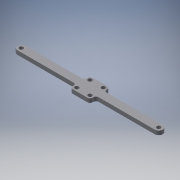
# Autodesk Inventor part: led_brace
Saved by Autodesk Inventor 2017 (Build 210142000, 142)
## iProperties
Created: 2017-06-15
Part Number: led_brace
Material: Generic
Document SubType Name: Modeling
Designer: millerid
Density: 1 g/cm^3
Appearance: Default
Author: millerid
Autodesk Inventor part; units mm, degrees
ref_plane "YZ Plane" through (0, 0, 0) normal (1, 0, 0) x (0, 1, 0)
ref_plane "XZ Plane" through (0, 0, 0) normal (0, 1, 0) x (-1, 0, 0)
ref_plane "XY Plane" through (0, 0, 0) normal (0, 0, 1) x (1, 0, 0)
sketch "Sketch1" plane through (0, 0, 0) normal (0, 1, 0) x (-1, 0, 0)
  circle A0 centre (13.6692, 0.0318) radius 1.5
  circle A1 centre (-89.8308, 0.0318) radius 1.5
  arc A2 (13.1692, -3) -> (14.1692, 2.9161) centre (13.6692, -0.042) ccw
  arc A3 (-89.8308, 3) -> (-89.8308, -3) centre (-89.8308, 0) ccw
  line L0 (-32.5808, -7.4682) -> (-43.5808, -7.4682)
  line L1 (-43.5808, 7.5318) -> (-32.5808, 7.5318)
  line L2 (13.1692, -3) -> (-28.5808, -3)
  line L3 (14.1692, 2.9161) -> (-28.5808, 2.9161)
  line L4 (-47.5808, -3) -> (-89.8308, -3)
  line L5 (-89.8308, 3) -> (-47.5808, 3)
  line L6 (-30.5808, -5.4682) -> (-30.5808, -5)
  line L7 (-30.5808, 4.9161) -> (-30.5808, 5.5318)
  line L8 (-45.5808, 5.5318) -> (-45.5808, 5)
  line L9 (-45.5808, -5) -> (-45.5808, -5.4682)
  circle A4 centre (-33.0808, -5.042) radius 1.5
  circle A5 centre (-43.0808, -5.042) radius 1.5
  circle A6 centre (-33.0808, 4.958) radius 1.5
  circle A7 centre (-43.0808, 4.958) radius 1.5
  arc A8 (-28.5808, -3) -> (-30.5808, -5) centre (-28.5808, -5) ccw
  arc A9 (-32.5808, -7.4682) -> (-30.5808, -5.4682) centre (-32.5808, -5.4682) ccw
  arc A10 (-45.5808, -5.4682) -> (-43.5808, -7.4682) centre (-43.5808, -5.4682) ccw
  arc A11 (-45.5808, -5) -> (-47.5808, -3) centre (-47.5808, -5) ccw
  arc A12 (-30.5808, 4.9161) -> (-28.5808, 2.9161) centre (-28.5808, 4.9161) ccw
  arc A13 (-47.5808, 3) -> (-45.5808, 5) centre (-47.5808, 5) ccw
  arc A14 (-43.5808, 7.5318) -> (-45.5808, 5.5318) centre (-43.5808, 5.5318) ccw
  arc A15 (-30.5808, 5.5318) -> (-32.5808, 7.5318) centre (-32.5808, 5.5318) ccw
  point P0 (-45.5808, 7.5318)
  point P1 (-45.5808, -7.4682)
  point P2 (-30.5808, 7.5318)
  dimension "d39" = 3
  dimension "d40" = 3
  dimension "d41" = 103.5
  dimension "d42" = 6
  dimension "d43" = 3
  dimension "d44" = 3
  dimension "d45" = 15
  dimension "d46" = 15
  dimension "d47" = 7.5
  dimension "d49" = 0
  dimension "d50" = 0
  dimension "d51" = 3
  dimension "d52" = 3
  dimension "d53" = 10
  dimension "d54" = 3
  dimension "d55" = 10
  dimension "d56" = 3
  dimension "d57" = 5
  dimension "d58" = 10
  dimension "d59" = 2
  dimension "d62" = 46.75
  dimension "d63" = 46.75
  dimension "d64" = 10
  dimension "d65" = 42.25
  constraints: 20 end point, 20 point on circle, 16 centre point, 16 tangent, 7 equal radius, 6 point on line, 4 collinear, 3 parallel, 2 horizontal, 1 vertical
  measures "d39" diameter of A0
  measures "d40" diameter of A1
  measures "d41" distance of A1.centre A0.centre
  measures "d42" distance of L2.start L3.start
  measures "d43" radius of A2
  measures "d44" radius of A3
  measures "d45" distance of point (-45.581, 7.532) point (-30.581, 7.532)
  measures "d46" distance of point (-45.581, -7.468) point (-45.581, 7.532)
  measures "d47" distance from line of A0.centre L0
  measures "d49" horizontal distance of A2.centre A0.centre
  measures "d50" horizontal distance of A3.centre A1.centre
  measures "d51" diameter of A4
  measures "d52" diameter of A5
  measures "d53" distance of A5.centre A4.centre
  measures "d54" diameter of A6
  measures "d55" distance of A6.centre A4.centre
  measures "d56" diameter of A7
  measures "d57" vertical distance of A2.centre A4.centre
  measures "d58" distance of A5.centre A7.centre
  measures "d59" radius of A8
  measures "d62" horizontal distance of A2.centre A4.centre
  measures "d63" horizontal distance of A0.centre A6.centre
  measures "d64" distance of A7.centre A6.centre
  measures "d65" horizontal distance of A3.centre A11.centre
extrude "Extrusion2" add sketch "Sketch1" along normal blind 3
equation "\"d47\" = 0.5 * d46"
equation "\"d55\" = d53"
equation "\"d57\" = 0.5 * d53"
equation "\"d58\" = d53"
equation "\"d62\" = -0.5 * d53 + 0.5 * d41"
equation "\"d63\" = d62"
equation "\"d64\" = d53"
body "Solid2"
